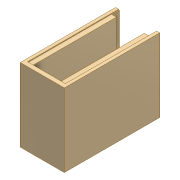
# Autodesk Inventor part: Reactor Bottom_v2
Saved by Autodesk Inventor 2016 (Build 200138000, 138)
## iProperties
Created: 2016-09-14
Part Number: Reactor Bottom_v2
Material: Polyethylene, Low Density
Document SubType Name: Modeling
Designer: jbui8
Density: 0.894 g/cm^3
Appearance: Smooth - Off-White
Author: jbui8
Autodesk Inventor part; units mm, degrees
ref_plane "XZ Plane" through (0, 0, 0) normal (0, 1, 0) x (-1, 0, 0)
sketch "Sketch1" plane through (0, 0, 0) normal (0, 0, 1) x (1, 0, 0)
  line L0 (0, 0) -> (30, 0)
  line L1 (30, 0) -> (30, 65)
  line L2 (30, 65) -> (0, 65)
  line L3 (0, 65) -> (0, 0)
  dimension "d0" = 30
  dimension "d1" = 65
  constraints: 8 end point, 2 parallel, 1 horizontal, 1 perpendicular
  measures "d0" distance of L2.end L1.end
  measures "d1" distance of L1.end L0.end
extrude "Extrusion1" add sketch "Sketch1" along normal blind 100
sketch "Sketch2" plane through (0, 0, 100) normal (0, 0, 1) x (1, 0, 0)
  line L0 (2.1, 2.877) -> (27.9, 2.877)
  line L1 (27.9, 2.877) -> (27.9, 68.621)
  line L2 (27.9, 68.621) -> (2.1, 68.621)
  line L3 (2.1, 68.621) -> (2.1, 2.877)
  line L4 (30, 65) -> (0, 65) construction
  line L5 (15, 65) -> (15, 0) construction
  line L6 (0, 0) -> (30, 0) construction
  dimension "d4" = 25.8
  constraints: 10 end point, 2 midpoint, 2 parallel, 1 horizontal, 1 perpendicular, 1 other
  measures "d4" distance of L2.end L1.end
extrude "Extrusion2" cut sketch "Sketch2" against normal blind 100
ref_plane "Work Plane1" through (0, 0, 50) normal (0, 0, 1) x (1, 0, 0)
sketch "Sketch3" plane through (0, 0, 50) normal (0, 0, 1) x (1, 0, 0)
  line L0 (2.1, 2.877) -> (27.9, 2.877) construction
  line L1 (15, 2.877) -> (15, 72.0179) construction
  line L2 (15, 65) -> (2.1, 65) construction
  line L3 (2.1, 65) -> (0, 65) construction
  line L4 (2.1, 65) -> (2.6, 65)
  line L5 (2.6, 65) -> (2.6, 60)
  line L6 (2.6, 60) -> (2.1, 60)
  line L7 (2.1, 60) -> (2.1, 65)
  line L8 (15, 60) -> (5.475, 60) construction
  line L9 (5.475, 60) -> (2.1, 60)
  line L10 (2.1, 60) -> (2.1, 2.877)
  line L11 (2.1, 2.877) -> (5.475, 2.877)
  line L12 (5.475, 2.877) -> (5.475, 60)
  point P0 (0, 0)
  dimension "d8" = 0.5
  dimension "d9" = 5
  dimension "d10" = 9.525
  constraints: 22 end point, 4 horizontal, 4 parallel, 2 collinear, 2 perpendicular, 2 point on line, 1 midpoint, 1 vertical
  measures "d8" distance of L5.end L6.end
  measures "d9" distance of L4.end L5.end
  measures "d10" distance of L8.start L8.end
extrude "Extrusion3" add sketch "Sketch3" along normal mid plane 99
ref_plane "Work Plane2" through (15, 0, 0) normal (1, 0, 0) x (0, 1, 0)
mirror "Mirror1" about plane through (15, 0, 0) normal (1, 0, 0) of "Extrusion3"
split "Split1" plane through (0, 0, 50) removes the side toward (0, 0, -1)
sketch "Sketch4" plane through (30, 0, 50) normal (0, 0, -1) x (-1, 0, 0)
  line L0 (27.9, 2.877) -> (27.9, 65) projected
  line L1 (2.1, 65) -> (2.1, 2.877) projected
  line L2 (27.9, 2.877) -> (2.1, 2.877)
  line L3 (2.1, 2.877) -> (2.1, 65)
  line L4 (2.1, 65) -> (27.9, 65)
  line L5 (27.9, 65) -> (27.9, 2.877)
  point P0 (30, 0)
  constraints: 8 end point, 2 parallel, 1 horizontal, 1 perpendicular
extrude "Extrusion4" cut sketch "Sketch4" against normal blind 0.5
body "Solid1"
